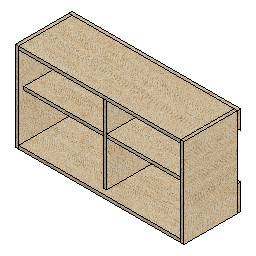
model (Autodesk Fusion 360 design; units mm, degrees)
Autodesk Fusion 360 part; units mm, degrees
sketch "Sketch1" plane through (0, 0, 0) normal (0, 1, 0) x (1, 0, 0)
  line L0 (0, 0) -> (945, 0)
  line L1 (945, 0) -> (945, -500)
  line L2 (945, -500) -> (0, -500)
  line L3 (0, -500) -> (0, 0)
  line L4 (18, -18) -> (927, -18)
  line L5 (927, -18) -> (927, -482)
  line L6 (927, -482) -> (18, -482)
  line L7 (18, -482) -> (18, -18)
  line L8 (18, -482) -> (18, -500)
  line L9 (927, -482) -> (927, -500)
  line L10 (927, -18) -> (927, 0)
  line L11 (18, -18) -> (18, 0)
  line L12 (463.5, -482) -> (463.5, -18)
  line L13 (481.5, -18) -> (481.5, -482)
  line L14 (463.5, -482) -> (472.5, -18) construction
  line L15 (472.5, -18) -> (481.5, -482) construction
  line L16 (18, -271) -> (463.5, -271)
  line L17 (18, -289) -> (463.5, -289)
  line L18 (472.5, -18) -> (472.5, 0) construction
  line L19 (927, -289) -> (481.5, -289)
  line L20 (927, -271) -> (481.5, -271)
  line L21 (0, -395) -> (945, -395)
  line L22 (795, 0) -> (795, -145)
  line L23 (795, -145) -> (945, -145)
  line L24 (0, -145) -> (150, -145)
  line L25 (150, -145) -> (150, 0)
  dimension "d1" = 945
  dimension "d2" = 500
  dimension "d4" = 18
  dimension "d5" = 18
  dimension "d6" = 18
  dimension "d7" = 253
  dimension "d16" = 105
  dimension "d17" = 150
  dimension "d18" = 145
  constraint horizontal L0
  constraint vertical L1
  constraint horizontal L2
  constraint vertical L3
  constraint coincident L0.start L3.end
  constraint coincident L2 L8.end
  constraint coincident L2 L9.end
  constraint coincident L0 L10.end
  constraint coincident L0 L11.end
  constraint vertical L11
  constraint vertical L8
  constraint vertical L9
  constraint vertical L10
  constraint coincident L6 L12.start
  constraint coincident L4 L12.end
  constraint coincident L4 L13.start
  constraint coincident L6 L13.end
  constraint vertical L12
  constraint vertical L13
  constraint midpoint L4 L14.end
  constraint equal L14 L15
  constraint coincident L7 L16.start
  constraint coincident L12 L16.end
  constraint coincident L7 L17.start
  constraint coincident L12 L17.end
  constraint horizontal L16
  constraint horizontal L17
  constraint midpoint L0 L18.end
  constraint symmetric L16.start L18 L20.start
  constraint symmetric L16.end L18 L20.end
  constraint symmetric L17.start L18 L19.start
  constraint symmetric L17.end L18 L19.end
  constraint coincident L3 L21.start
  constraint coincident L1 L21.end
  constraint coincident L0 L22.start
  constraint coincident L1 L23.end
  constraint coincident L3 L24.start
  constraint coincident L0 L25.end
  constraint horizontal L24
  constraint vertical L25
  constraint horizontal L21
  constraint vertical L22
  constraint horizontal L23
  constraint equal L23 L24
  constraint equal L22 L25
  measures "d1" distance of L0.start L0.end
  measures "d2" distance of L0.start L2.end
  measures "d5" distance of L12.end L13.start
  measures "d6" distance of L16.start L17.start
  measures "d7" distance of L4.start L16.start
  measures "d16" distance of L2.end L21.start
  measures "d17" distance of L0.start L25.end
  measures "d18" distance of L0.start L24.start
extrude "Extrude1" add sketch "Sketch1" against normal blind 300 contours L0 L3 L7 L11 L24 | L3 L7 L21 L24 | L2 L3 L7 L8 L21 | L0 L1 L5 L10 L23 | L1 L2 L5 L9 L21 | L1 L5 L21 L23 makes body 1 at (0, -200, 333.3333) makes body 2 at (927, -200, 333.3333)
extrude "Extrude2" add sketch "Sketch1" against normal up to surface (300 mm away) separate body contours L0 L4 L11 L25 | L0 L4 L22 L25 | L0 L4 L10 L22 | L2 L6 L8 L9 makes body 3 at (624, -100, 482) makes body 4 at (321, -200, 0)
extrude "Extrude3" add sketch "Sketch1" against normal blind 270 separate body contours L4 L12 L13 L21 | L6 L12 L13 L21 makes body 5
extrude "Extrude4" add sketch "Sketch1" against normal up to surface (270 mm away) separate body contours L7 L12 L16 L17 | L5 L13 L19 L20 makes body 6 at (166.5, -90, 271) makes body 7 at (778.5, -90, 271)
extrude "Extrude5" add sketch "Sketch1" along normal blind 18 separate body contours L0 L3 L7 L11 L24 | L0 L4 L11 L25 | L4 L7 L24 L25 | L2 L3 L7 L8 L21 | L0 L4 L10 L22 | L6 L7 L12 L21 | L0 L1 L5 L10 L23 | L4 L5 L22 L23 | L2 L6 L8 L9 | L6 L12 L13 L21 | L1 L2 L5 L9 L21 | L5 L6 L13 L21 makes body 8 at (315, 0, 465) makes body 9 at (845, 0, 96.6667) makes body 10 at (100, 0, 48.3333)
chamfer "Chamfer1" distance 18 angle 45 1 edges at (472.5, 0, 395) on bodies 8
sketch "Sketch2" plane through (18, 0, 0) normal (1, 0, 0) x (0, 1, 0)
  line L0 (0, 0) -> (0, 500)
  line L1 (0, 500) -> (-300, 500)
  line L2 (-300, 500) -> (-300, 0)
  line L3 (-300, 0) -> (0, 0)
  line L4 (-270, 289) -> (-270, 271)
  line L5 (-270, 271) -> (0, 271)
  line L6 (0, 271) -> (0, 289)
  line L7 (0, 289) -> (-270, 289)
  circle A0 centre (-233, 268) radius 3
  circle A1 centre (-37, 268) radius 3
  dimension "d22" = 37
  dimension "d24" = 37
  dimension "d25" = 6
  dimension "d26" = 6
  constraint tangent L5 A0
  constraint tangent L5 A1
  measures "d22" horizontal distance of L5.end A1.centre
  measures "d24" horizontal distance of L4.end A0.centre
  measures "d25" diameter of A1
  measures "d26" diameter of A0
extrude "Extrude6" cut sketch "Sketch2" along normal up to surface (929 mm away) from surface at -10 contours A1 | A0 bodies 1 2 5
extrude "Extrude7" add 2 faces at (8, -37.8262, 267.1386) (8, -233.6235, 268.7818) along direction (1, 0, 0) blind 60 separate body on bodies 1 makes body 11 at (48, -38.9851, 265.7507) makes body 12 at (48, -234.9851, 265.7507)
extrude "Extrude8" add sketch "Sketch2" along normal up to surface (60 mm away) from surface at 424.5 separate body contours A1 | A0 makes body 13 at (482.5, -231.0149, 270.2493) makes body 14 at (482.5, -39.0947, 270.1476)
chamfer "Chamfer2" distance 2 distance2 1 6 edges at (68, -235.797, 266.9152) (68, -39.797, 266.9152) (442.5, -235.797, 266.9152) (502.5, -235.797, 269.0848) (442.5, -39.797, 266.9152) (502.5, -39.797, 269.0848) measured on face at (68, -233.6235, 268.7818) measured on face at (68, -37.8262, 267.1386) measured on face at (482.5, -231.0149, 270.2493) measured on face at (482.5, -231.0149, 270.2493) measured on face at (482.5, -39.0947, 270.1476) measured on face at (482.5, -39.0947, 270.1476) on bodies 11 12 13 14
ref_plane "WorkPlane1" through (472.5, -135, 250) normal (-1, 0, 0) x (0, 0, -1)
mirror "Mirror1" about plane through (472.5, -135, 250) normal (-1, 0, 0) of bodies 12 11 makes body 15 at (897.6667, -38.9851, 265.7507) makes body 16 at (897.6667, -234.9851, 265.7507)
equation "th = 18 mm"
equation "d4 = th"
equation "d5 = th"
equation "d6 = th"
equation "d7 = 250 mm + 3 mm"
equation "d19 = th"
equation "d21 = th"
equation "d24 = d22"
equation "d26 = d25"
equation "d32 = ( ( 60 - 18 ) / 2 ) * 1 mm"
equation "d33 = ( ( 60 - 18 ) / 2 ) * 1 mm"
